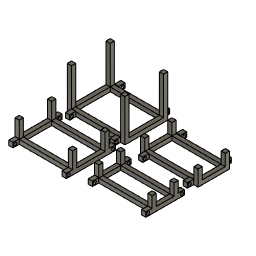
OpenDesgin_Moch-up v5 (Autodesk Fusion 360 design; units mm, degrees)
Autodesk Fusion 360 part; units mm, degrees
sketch "スケッチ1" plane through (0, 0, 0) normal (0, 0, 1) x (1, 0, 0)
  line L0 (27.5, -17.5) -> (-27.5, -17.5)
  line L1 (-27.5, -17.5) -> (-27.5, 17.5)
  line L2 (-27.5, 17.5) -> (27.5, 17.5)
  line L3 (27.5, 17.5) -> (27.5, -17.5)
  line L4 (27.5, -17.5) -> (-27.5, 17.5) construction
  line L5 (-27.5, -17.5) -> (27.5, 17.5) construction
  line L6 (27.5, -52.5) -> (-27.5, -22.5) construction
  line L7 (-27.5, -52.5) -> (27.5, -22.5) construction
  line L8 (-27.5, -52.5) -> (-27.5, -22.5)
  line L9 (-27.5, -22.5) -> (27.5, -22.5)
  line L10 (27.5, -52.5) -> (-27.5, -52.5)
  line L11 (27.5, -22.5) -> (27.5, -52.5)
  line L12 (0, 0) -> (0, -37.5) construction
  line L13 (-27.5, -82.5) -> (-27.5, -57.5)
  line L14 (-27.5, -57.5) -> (27.5, -57.5)
  line L15 (27.5, -57.5) -> (27.5, -82.5)
  line L16 (-27.5, -82.5) -> (27.5, -57.5) construction
  line L17 (27.5, -82.5) -> (-27.5, -57.5) construction
  line L18 (27.5, -82.5) -> (-27.5, -82.5)
  line L19 (27.5, 22.5) -> (-27.5, 63.5) construction
  line L20 (0, 43) -> (0, -6.9722) construction
  line L21 (-27.5, 22.5) -> (-27.5, 63.5)
  line L22 (-27.5, 22.5) -> (27.5, 63.5) construction
  line L23 (-27.5, 63.5) -> (27.5, 63.5)
  line L24 (27.5, 22.5) -> (-27.5, 22.5)
  line L25 (27.5, 63.5) -> (27.5, 22.5)
  line L26 (23.5, 26.5) -> (-23.5, 26.5)
  line L27 (-23.5, 26.5) -> (-23.5, 59.5)
  line L28 (-23.5, 59.5) -> (23.5, 59.5)
  line L29 (23.5, 59.5) -> (23.5, 26.5)
  line L30 (23.5, 26.5) -> (-23.5, 59.5) construction
  line L31 (-23.5, 26.5) -> (23.5, 59.5) construction
  line L32 (23.5, -13.5) -> (-23.5, -13.5)
  line L33 (-23.5, -13.5) -> (-23.5, 13.5)
  line L34 (-23.5, 13.5) -> (23.5, 13.5)
  line L35 (23.5, 13.5) -> (23.5, -13.5)
  line L36 (23.5, -13.5) -> (-23.5, 13.5) construction
  line L37 (-23.5, -13.5) -> (23.5, 13.5) construction
  line L38 (23.5, -48.5) -> (-23.5, -48.5)
  line L39 (-23.5, -48.5) -> (-23.5, -26.5)
  line L40 (-23.5, -26.5) -> (23.5, -26.5)
  line L41 (23.5, -26.5) -> (23.5, -48.5)
  line L42 (23.5, -48.5) -> (-23.5, -26.5) construction
  line L43 (-23.5, -48.5) -> (23.5, -26.5) construction
  line L44 (23.5, -78.5) -> (-23.5, -78.5)
  line L45 (-23.5, -78.5) -> (-23.5, -61.5)
  line L46 (-23.5, -61.5) -> (23.5, -61.5)
  line L47 (23.5, -61.5) -> (23.5, -78.5)
  line L48 (23.5, -78.5) -> (-23.5, -61.5) construction
  line L49 (-23.5, -78.5) -> (23.5, -61.5) construction
  line L50 (-27.5, 63.5) -> (-23.5, 63.5)
  line L51 (-23.5, 63.5) -> (-23.5, 59.5)
  line L52 (-23.5, 59.5) -> (-27.5, 59.5)
  line L53 (-27.5, 59.5) -> (-27.5, 63.5)
  line L54 (27.5, 63.5) -> (23.5, 63.5)
  line L55 (23.5, 63.5) -> (23.5, 59.5)
  line L56 (23.5, 59.5) -> (27.5, 59.5)
  line L57 (27.5, 59.5) -> (27.5, 63.5)
  line L58 (27.5, 22.5) -> (23.5, 22.5)
  line L59 (23.5, 22.5) -> (23.5, 26.5)
  line L60 (23.5, 26.5) -> (27.5, 26.5)
  line L61 (27.5, 26.5) -> (27.5, 22.5)
  line L62 (-27.5, 22.5) -> (-23.5, 22.5)
  line L63 (-23.5, 22.5) -> (-23.5, 26.5)
  line L64 (-23.5, 26.5) -> (-27.5, 26.5)
  line L65 (-27.5, 26.5) -> (-27.5, 22.5)
  line L66 (-27.5, -17.5) -> (-23.5, -17.5)
  line L67 (-23.5, -17.5) -> (-23.5, -13.5)
  line L68 (-23.5, -13.5) -> (-27.5, -13.5)
  line L69 (-27.5, -13.5) -> (-27.5, -17.5)
  line L70 (-27.5, 17.5) -> (-23.5, 17.5)
  line L71 (-23.5, 17.5) -> (-23.5, 13.5)
  line L72 (-23.5, 13.5) -> (-27.5, 13.5)
  line L73 (-27.5, 13.5) -> (-27.5, 17.5)
  line L74 (27.5, 17.5) -> (23.5, 17.5)
  line L75 (23.5, 17.5) -> (23.5, 13.5)
  line L76 (23.5, 13.5) -> (27.5, 13.5)
  line L77 (27.5, 13.5) -> (27.5, 17.5)
  line L78 (27.5, -17.5) -> (23.5, -17.5)
  line L79 (23.5, -17.5) -> (23.5, -13.5)
  line L80 (23.5, -13.5) -> (27.5, -13.5)
  line L81 (27.5, -13.5) -> (27.5, -17.5)
  line L82 (27.5, -52.5) -> (23.5, -52.5)
  line L83 (23.5, -52.5) -> (23.5, -48.5)
  line L84 (23.5, -48.5) -> (27.5, -48.5)
  line L85 (27.5, -48.5) -> (27.5, -52.5)
  line L86 (27.5, -22.5) -> (23.5, -22.5)
  line L87 (23.5, -22.5) -> (23.5, -26.5)
  line L88 (23.5, -26.5) -> (27.5, -26.5)
  line L89 (27.5, -26.5) -> (27.5, -22.5)
  line L90 (-27.5, -22.5) -> (-23.5, -22.5)
  line L91 (-23.5, -22.5) -> (-23.5, -26.5)
  line L92 (-23.5, -26.5) -> (-27.5, -26.5)
  line L93 (-27.5, -26.5) -> (-27.5, -22.5)
  line L94 (-27.5, -52.5) -> (-23.5, -52.5)
  line L95 (-23.5, -52.5) -> (-23.5, -48.5)
  line L96 (-23.5, -48.5) -> (-27.5, -48.5)
  line L97 (-27.5, -48.5) -> (-27.5, -52.5)
  line L98 (-27.5, -57.5) -> (-23.5, -57.5)
  line L99 (-23.5, -57.5) -> (-23.5, -61.5)
  line L100 (-23.5, -61.5) -> (-27.5, -61.5)
  line L101 (-27.5, -61.5) -> (-27.5, -57.5)
  line L102 (-27.5, -82.5) -> (-23.5, -82.5)
  line L103 (-23.5, -82.5) -> (-23.5, -78.5)
  line L104 (-23.5, -78.5) -> (-27.5, -78.5)
  line L105 (-27.5, -78.5) -> (-27.5, -82.5)
  line L106 (27.5, -82.5) -> (23.5, -82.5)
  line L107 (23.5, -82.5) -> (23.5, -78.5)
  line L108 (23.5, -78.5) -> (27.5, -78.5)
  line L109 (27.5, -78.5) -> (27.5, -82.5)
  line L110 (27.5, -57.5) -> (23.5, -57.5)
  line L111 (23.5, -57.5) -> (23.5, -61.5)
  line L112 (23.5, -61.5) -> (27.5, -61.5)
  line L113 (27.5, -61.5) -> (27.5, -57.5)
  point P0 (0, -37.5)
  point P1 (0, -37.5)
  point P2 (0, -70)
  point P3 (0, -70)
  point P4 (0, -70)
  point P5 (0, 43)
  point P6 (0, 43)
  point P7 (0, 43)
  point P8 (0, -37.5)
  point P9 (0, -70)
  dimension "d1" = 55
  dimension "d2" = 35
  dimension "d3" = 55
  dimension "d4" = 30
  dimension "d5" = 5
  dimension "d6" = 90
  dimension "d7" = 55
  dimension "d8" = 25
  dimension "d9" = 5
  dimension "d10" = 55
  dimension "d11" = 41
  dimension "d12" = 90
  dimension "d13" = 5
  dimension "d14" = 4
  dimension "d15" = 4
  dimension "d16" = 4
  dimension "d17" = 4
  dimension "d18" = 4
  dimension "d20" = 4
  dimension "d21" = 4
  dimension "d22" = 4
  constraint horizontal L0
  constraint perpendicular L0 L1
  constraint parallel L0 L2
  constraint parallel L1 L3
  constraint coincident L4 L12.start
  constraint coincident L5 L12.start
  constraint coincident L12.start origin
  constraint horizontal L10
  constraint perpendicular L8 L10
  constraint parallel L9 L10
  constraint parallel L8 L11
  constraint coincident P8 L6
  constraint coincident P8 L7
  constraint coincident P8 P1
  constraint horizontal L18
  constraint perpendicular L13 L18
  constraint parallel L14 L18
  constraint parallel L13 L15
  constraint coincident P9 L17
  constraint coincident P9 L16
  constraint coincident P9 P4
  constraint collinear L11 L15
  constraint horizontal L24
  constraint perpendicular L21 L24
  constraint parallel L23 L24
  constraint parallel L21 L25
  constraint coincident P7 L19
  constraint coincident P7 L22
  constraint coincident P7 P6
  constraint collinear L3 L25
  constraint horizontal L26
  constraint perpendicular L26 L27
  constraint parallel L26 L28
  constraint parallel L27 L29
  constraint coincident L30 P7
  constraint coincident L31 P7
  constraint horizontal L32
  constraint perpendicular L32 L33
  constraint parallel L32 L34
  constraint parallel L33 L35
  constraint coincident L36 L12.start
  constraint coincident L37 L12.start
  constraint horizontal L38
  constraint perpendicular L38 L39
  constraint parallel L38 L40
  constraint parallel L39 L41
  constraint coincident L42 P8
  constraint coincident L43 P8
  constraint horizontal L44
  constraint perpendicular L44 L45
  constraint parallel L44 L46
  constraint parallel L45 L47
  constraint coincident L48 P9
  constraint coincident L49 P9
  constraint horizontal L50
  constraint vertical L51
  constraint horizontal L52
  constraint vertical L53
  constraint horizontal L54
  constraint vertical L55
  constraint horizontal L56
  constraint vertical L57
  constraint horizontal L58
  constraint vertical L59
  constraint horizontal L60
  constraint vertical L61
  constraint horizontal L62
  constraint vertical L63
  constraint horizontal L64
  constraint vertical L65
  constraint horizontal L66
  constraint vertical L67
  constraint horizontal L68
  constraint vertical L69
  constraint horizontal L70
  constraint vertical L71
  constraint horizontal L72
  constraint vertical L73
  constraint horizontal L74
  constraint vertical L75
  constraint horizontal L76
  constraint vertical L77
  constraint horizontal L78
  constraint vertical L79
  constraint horizontal L80
  constraint vertical L81
  constraint horizontal L82
  constraint vertical L83
  constraint horizontal L84
  constraint vertical L85
  constraint horizontal L86
  constraint vertical L87
  constraint horizontal L88
  constraint vertical L89
  constraint horizontal L90
  constraint vertical L91
  constraint horizontal L92
  constraint vertical L93
  constraint horizontal L94
  constraint vertical L95
  constraint horizontal L96
  constraint vertical L97
  constraint horizontal L98
  constraint vertical L99
  constraint horizontal L100
  constraint vertical L101
  constraint horizontal L102
  constraint vertical L103
  constraint horizontal L104
  constraint vertical L105
  constraint horizontal L106
  constraint vertical L107
  constraint horizontal L108
  constraint vertical L109
  constraint horizontal L110
  constraint vertical L111
  constraint horizontal L112
  constraint vertical L113
  measures "d1" distance of L1.end L2.end
  measures "d2" distance of L0.start L2.end
  measures "d3" distance of L6.end L7.end
  measures "d4" distance of L6.start L7.end
  measures "d5" distance of L0 L9
  measures "d6" angle of L2 L12
  measures "d7" distance of L14.end L13.end
  measures "d8" distance of L14.end L15.end
  measures "d9" distance of L10 L14
  measures "d10" distance of L19.end L22.end
  measures "d11" distance of L19.start L22.end
  measures "d12" angle of L20 L23
  measures "d13" distance of L2 L24
  measures "d14" distance of L15 L47
  measures "d15" distance of L18 L44
  measures "d16" distance of L11 L41
  measures "d17" distance of L10 L38
  measures "d18" distance of L3 L35
  measures "d20" distance of L0 L32
  measures "d21" distance of L24 L26
  measures "d22" distance of L21 L27
extrude "押し出し1" add sketch "スケッチ1" along normal blind 4 contours L21 L24 L62 L63 L64 L65 | L21 L27 L52 L64 | L24 L26 L59 L63 | L21 L23 L50 L51 L52 L53 | L24 L25 L58 L59 L60 L61 | L23 L28 L51 L55 | L25 L29 L56 L60 | L23 L25 L54 L55 L56 L57 makes body 1
extrude "押し出し2" add sketch "スケッチ1" along normal blind 4 separate body contours L0 L3 L78 L79 L80 L81 | L0 L32 L67 L79 | L3 L35 L76 L80 | L0 L1 L66 L67 L68 L69 | L2 L3 L74 L75 L76 L77 | L1 L33 L68 L72 | L2 L34 L71 L75 | L1 L2 L70 L71 L72 L73 | L8 L10 L94 L95 L96 L97 | L8 L39 L92 L96 | L10 L38 L83 L95 | L8 L9 L90 L91 L92 L93 | L10 L11 L82 L83 L84 L85 | L9 L40 L87 L91 | L11 L41 L84 L88 | L9 L11 L86 L87 L88 L89 | L13 L18 L102 L103 L104 L105 | L13 L45 L100 L104 | L18 L44 L103 L107 | L13 L14 L98 L99 L100 L101 | L15 L18 L106 L107 L108 L109 | L14 L46 L99 L111 | L15 L47 L108 L112 | L14 L15 L110 L111 L112 L113 makes body 2 at (-7.8333, 16.1667, 0) makes body 3 at (-7.8333, -23.8333, 0) makes body 4 at (7.8333, -81.1667, 0)
extrude "押し出し3" add sketch "スケッチ1" along normal blind 15 contours L8 L10 L94 L95 L96 L97 | L8 L9 L90 L91 L92 L93 | L10 L11 L82 L83 L84 L85 | L9 L11 L86 L87 L88 L89 | L13 L18 L102 L103 L104 L105 | L13 L14 L98 L99 L100 L101 | L15 L18 L106 L107 L108 L109 | L14 L15 L110 L111 L112 L113 bodies 3 4
extrude "押し出し4" add sketch "スケッチ1" along normal blind 20 contours L0 L3 L78 L79 L80 L81 | L0 L1 L66 L67 L68 L69 | L2 L3 L74 L75 L76 L77 | L1 L2 L70 L71 L72 L73 bodies 2
extrude "押し出し5" add sketch "スケッチ1" along normal blind 40 contours L21 L24 L62 L63 L64 L65 | L21 L23 L50 L51 L52 L53 | L24 L25 L58 L59 L60 L61 | L23 L25 L54 L55 L56 L57 bodies 1
sketch "スケッチ2" plane through (0, 0, 0) normal (0, 1, 0) x (1, 0, 0)
  line L0 (0, 0) -> (4.5, 0)
  line L1 (4.5, 0) -> (4.5, -4.5)
  line L2 (4.5, -4.5) -> (0, -4.5)
  line L3 (0, -4.5) -> (0, 0)
  line L4 (2.25, -2.25) -> (2.25, 0) construction
  circle A0 centre (2.25, -2.25) radius 1.5
  circle A1 centre (8.25, -2.25) radius 1.65
  line L5 (10.5, 0) -> (10.5, -4.5)
  line L6 (6, -4.5) -> (6, 0)
  line L7 (8.25, -2.25) -> (8.25, 0) construction
  line L8 (10.5, -4.5) -> (6, -4.5)
  line L9 (10.5, 0) -> (6, 0)
  dimension "d33" = 4.5
  dimension "d34" = 4.5
  dimension "d35" = 3
  dimension "d36" = 4.5
  dimension "d37" = 4.5
  dimension "d38" = 3.3
  constraint horizontal L0
  constraint vertical L1
  constraint horizontal L2
  constraint vertical L3
  constraint coincident L0.start L3.end
  constraint midpoint L0 L4.end
  constraint perpendicular L0 L4
  constraint coincident L4.start A0.centre
  constraint vertical L5
  constraint horizontal L8
  constraint vertical L6
  constraint coincident A1.centre L7.start
  constraint perpendicular L6 L9
  measures "d33" distance of L0.start L2.end
  measures "d34" distance of L1.end L2.end
  measures "d35" diameter of A0
  measures "d36" distance of L6.end L6.start
  measures "d37" distance of L5.end L6.start
  measures "d38" diameter of A1
extrude "押し出し6" add sketch "スケッチ2" against normal blind 4 separate body makes body 5 at (9.8979, -2.6667, 2.3322) makes body 6 at (3.7481, -2.6667, 2.3248)
copy_body "ボディのコピーと貼り付け1" bodies 6 makes body 7
move_body "移動1" bodies 7 to x (0, 1, 0) y (-1, 0, 0) z (0, 0, 1) at (23.5, -89, 0)
copy_body "ボディのコピーと貼り付け2" bodies 7 makes body 8
move_body "移動2" bodies 8 to x (1, 0, 0) y (0, 1, 0) z (0, 0, 1) at (-51, 0, 0)
copy_body "ボディのコピーと貼り付け3" bodies 7 8 makes body 9 makes body 10
move_body "移動3" bodies 9 10 to x (1, 0, 0) y (0, 1, 0) z (0, 0, 1) at (0, 33, 0)
move_body "移動4" bodies 4 10 9 8 7 to x (1, 0, 0) y (0, 1, 0) z (0, 0, 1) at (0, -5, 0)
move_body "移動5" bodies 7 to x (1, 0, 0) y (0, 1, 0) z (0, 0, 1) at (0, 0.5, 0)
move_body "移動6" bodies 8 to x (1, 0, 0) y (0, 1, 0) z (0, 0, 1) at (0, 0.5, 0)
extrude "押し出し7" add 2 faces at (24.8333, -61, 3) (-26.1667, -61, 3) along direction (0, -1, 0) blind 1.5 on bodies 9 10 bodies 9 4 10
move_body "移動7" bodies 9 8 7 to x (1, 0, 0) y (0, 1, 0) z (0, 0, 1) at (0, -34, 0)
copy_body "ボディのコピーと貼り付け4" bodies 8 7 makes body 11 makes body 12
move_body "移動8" bodies 11 12 to x (1, 0, 0) y (0, 1, 0) z (0, 0, 1) at (0, 69, 0)
move_body "移動9" bodies 11 12 3 to x (1, 0, 0) y (0, 1, 0) z (0, 0, 1) at (0, -25, 0)
move_body "移動10" bodies 11 to x (1, 0, 0) y (0, 1, 0) z (0, 0, 1) at (4.2, 0, 0)
move_body "移動11" bodies 12 to x (1, 0, 0) y (0, 1, 0) z (0, 0, 1) at (-4.2, 0, 0)
copy_body "ボディのコピーと貼り付け5" bodies 11 12 makes body 13 makes body 14
move_body "移動12" bodies 13 14 to x (1, 0, 0) y (0, 1, 0) z (0, 0, 1) at (0, 38, 0)
move_body "移動13" bodies 14 13 to x (1, 0, 0) y (0, 1, 0) z (0, 0, 1) at (0, -0.5, 0)
copy_body "ボディのコピーと貼り付け6" bodies 14 13 makes body 15 makes body 16
move_body "移動14" bodies 15 16 to x (1, 0, 0) y (0, 1, 0) z (0, 0, 1) at (0, 10, 0)
move_body "移動15" bodies 1 to x (1, 0, 0) y (0, 1, 0) z (0, 0, 1) at (0, 10, 0)
move_body "移動16" bodies 16 15 to x (1, 0, 0) y (0, 1, 0) z (0, 0, 1) at (0, 60, 0)
move_body "移動17" bodies 15 16 to x (1, 0, 0) y (0, 1, 0) z (0, 0, 1) at (0, 1.5, 0)
copy_body "ボディのコピーと貼り付け7" bodies 7 8 makes body 17 makes body 18
move_body "移動18" bodies 17 18 to x (1, 0, 0) y (0, 1, 0) z (0, 0, 1) at (0, 110, 0)
move_body "移動19" bodies 17 18 to x (1, 0, 0) y (0, 1, 0) z (0, 0, 1) at (0, -6, 0)
copy_body "ボディのコピーと貼り付け8" bodies 18 17 makes body 19 makes body 20
move_body "移動20" bodies 19 20 to x (1, 0, 0) y (0, 1, 0) z (0, 0, 1) at (0, 41, 0)
move_body "移動21" bodies 19 20 to x (1, 0, 0) y (0, 1, 0) z (0, 0, 1) at (0, 2, 0)
move_body "移動22" bodies 19 20 to x (1, 0, 0) y (0, 1, 0) z (0, 0, 1) at (0, -0.5, 0)
move_body "移動23" bodies 16 15 to x (1, 0, 0) y (0, 1, 0) z (0, 0, 1) at (0, 1, 0)
copy_body "ボディのコピーと貼り付け9" bodies 15 16 makes body 21 makes body 22
move_body "移動24" bodies 21 22 to x (1, 0, 0) y (0, 1, 0) z (0, 0, 1) at (0, 48.5, 0)
extrude "押し出し8" add 2 faces at (-21.9667, 75, 3) (20.6333, 75, 3) along direction (0, -1, 0) blind 1.5 on bodies 21 22 bodies 22 1 21
extrude "押し出し9" add 2 faces at (-21.9667, 31, 1.5) (20.6333, 31, 1.5) along direction (0, 1, 0) blind 1.5 on bodies 15 16 bodies 16 15 22
extrude "押し出し10" add 2 faces at (-26.1667, 19, 3) (24.8333, 19, 3) along direction (0, -1, 0) blind 1.5 on bodies 19 20 bodies 19 2 20
extrude "押し出し11" add 2 faces at (24.8333, -19, 1.5) (-26.1667, -19, 1.5) along direction (0, 1, 0) blind 1.5 on bodies 17 18 bodies 17 18 19
extrude "押し出し12" add 2 faces at (20.6333, -46, 3) (-21.9667, -46, 3) along direction (0, -1, 0) blind 1.5 on bodies 13 14 bodies 14 3 13
extrude "押し出し13" add 2 faces at (-26.1667, -123, 1.5) (24.8333, -123, 1.5) along direction (0, 1, 0) blind 1.5 on bodies 7 8 bodies 8 7 9
extrude "押し出し14" add 2 faces at (-21.9667, -79, 1.5) (20.6333, -79, 1.5) along direction (0, 1, 0) blind 1.5 on bodies 11 12 bodies 11 12 14
move_body "移動25" bodies 11 8 to x (1, 0, 0) y (0, 1, 0) z (0, 0, 1) at (70, 110, 0)
hidden bodies 5 6
